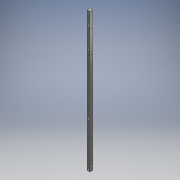
# Autodesk Inventor part: longitudinal
Saved by Autodesk Inventor 2016 (Build 200138000, 138)
## iProperties
Created: 2015-10-11
Part Number: longitudinal
Material: Aluminum
Document SubType Name: Modeling
Designer: Artur
Density: 2.7 g/cm^3
Appearance: Satin
Mass: 60.1938 g
Surface Area: 51.84 cm^2
Volume: 7.668 cm^3
Author: Artur
Autodesk Inventor part; units mm, degrees
ref_plane "YZ Plane" through (0, 0, 0) normal (1, 0, 0) x (0, 1, 0)
ref_plane "XZ Plane" through (0, 0, 0) normal (0, 1, 0) x (-1, 0, 0)
ref_plane "XY Plane" through (0, 0, 0) normal (0, 0, 1) x (1, 0, 0)
sketch "Sketch1" plane through (0, 0, 0) normal (0, 0, 1) x (1, 0, 0)
  line L0 (0, 6) -> (6, 6)
  line L1 (6, 6) -> (6, 0)
  line L2 (6, 0) -> (0, 0)
  line L3 (0, 0) -> (0, 6)
  dimension "d0" = 6
  dimension "d1" = 6
  constraints: 8 end point, 2 parallel, 1 coincident, 1 horizontal, 1 perpendicular
  measures "d0" distance of L1.end L2.end
  measures "d1" distance of L0.end L1.end
extrude "Extrusion1" add sketch "Sketch1" along normal blind 300
sketch "Sketch3" plane through (0, 0, 0) normal (0, 1, 0) x (-1, 0, 0)
  line L0 (-6, 300) -> (0, 300) construction
  line L1 (-6, 0) -> (-6, 300) construction
  line L2 (0, 0) -> (0, 300) construction
  line L3 (0, 0) -> (-6, 0) construction
  line L4 (-3, 0) -> (-3, 300) construction
  line L5 (0, 300) -> (-6, 300) projected
  line L6 (-6, 0) -> (0, 0) projected
  point P0 (-3, 227)
  point P1 (-3, 98)
  point P2 (-3, 272)
  point P3 (-3, 3)
  dimension "d8" = 129
  dimension "d17" = 73
  dimension "d18" = 28
  dimension "d19" = 3
  constraints: 10 end point, 4 midpoint, 4 point on line
  measures "d8" distance of point (-3, 98) point (-3, 227)
  measures "d17" distance of L4.end point (-3, 227)
  measures "d18" distance from line of L0 point (-3, 272)
  measures "d19" distance from line of L6 point (-3, 3)
hole "Hole1" at (3, 0, 227) at (3, 0, 98) at (3, 0, 3) at (3, 0, 272) direction (0, 1, 0) diameter 3 end through all
sketch "Sketch4" plane through (0, 0, 0) normal (-1, 0, 0) x (0, 0, 1)
  line L0 (0, 0) -> (0, 6) construction
  line L1 (0, 0) -> (300, 0) construction
  line L2 (300, 6) -> (300, 0) construction
  line L3 (0, 6) -> (300, 6) construction
  line L4 (0, 0) -> (0, 6) construction
  line L5 (0, 3) -> (300, 3) construction
  line L6 (300, 6) -> (300, 0) construction
  point P0 (266, 3)
  point P1 (9, 3)
  dimension "d20" = 9
  dimension "d21" = 34
  constraints: 2 end point, 2 midpoint, 2 point on line
  measures "d20" distance from line of point (9, 3) L0
  measures "d21" distance from line of point (266, 3) L2
hole "Hole2" at (0, 3, 266) at (0, 3, 9) direction (1, 0, 0) diameter 3 end through all
equation "\"d1\" = d0"
body "Solid1"
